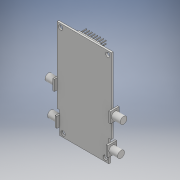
# Autodesk Inventor part: PE-43120-EVB
Saved by Autodesk Inventor 2018 (Build 220112000, 112)
## iProperties
Created: 2018-01-02
Part Number: PE-43120-EVB
Material: Generic
Document SubType Name: Modeling
Designer: rwradema
Density: 1 g/cm^3
Appearance: Default
Author: rwradema
Autodesk Inventor part; units mm, degrees
ref_plane "YZ Plane" through (0, 0, 0) normal (1, 0, 0) x (0, 1, 0)
ref_plane "XZ Plane" through (0, 0, 0) normal (0, 1, 0) x (-1, 0, 0)
ref_plane "XY Plane" through (0, 0, 0) normal (0, 0, 1) x (1, 0, 0)
sketch "Sketch1" plane through (0, 0, 0) normal (0, 1, 0) x (-1, 0, 0)
  line L0 (24.8, -18.7) -> (24.8, 50)
  line L1 (24.8, 50) -> (-24.8, 50)
  line L2 (-24.8, 50) -> (-24.8, -18.7)
  line L3 (-24.8, -18.7) -> (-22.5, -18.7)
  line L4 (-22.5, -18.7) -> (-22.5, -39)
  line L5 (-22.5, -39) -> (22.5, -39)
  line L6 (22.5, -39) -> (22.5, -18.7)
  line L7 (22.5, -18.7) -> (24.8, -18.7)
  line L8 (0, 42.3382) -> (0, -37.7046) construction
  point P0 (0, 0)
  dimension "d0" = 49.6
  dimension "d1" = 45
  dimension "d2" = 89
  dimension "d3" = 68.7
  dimension "d4" = 50
  constraints: 18 end point, 8 perpendicular, 1 collinear, 1 point on line, 1 vertical, 1 other
  measures "d0" distance of L0.end L1.end
  measures "d1" distance of L4.end L5.end
  measures "d2" distance between parallel lines of L1 L5
  measures "d3" distance of L0.start L0.end
  measures "d4" distance from line of L1 point (0, 0)
extrude "Extrusion1" add sketch "Sketch1" along normal blind 1.63
sketch "Sketch2" plane through (0, 1.63, 0) normal (0, 1, 0) x (1, 0, 0)
  circle A0 centre (-21.55, -46.75) radius 2
  circle A1 centre (21.55, -46.75) radius 2
  circle A2 centre (19.25, 35.75) radius 2
  circle A3 centre (-19.25, 35.75) radius 2
  line L0 (-24.8, 18.7) -> (-24.8, -50) projected
  line L1 (-24.8, -50) -> (24.8, -50) projected
  line L2 (22.5, 39) -> (-22.5, 39) projected
  line L3 (22.5, 18.7) -> (22.5, 39) projected
  line L4 (-22.5, 39) -> (-22.5, 18.7) projected
  point P0 (0, 0)
  dimension "d7" = 4
  dimension "d8" = 3.25
  dimension "d9" = 3.25
  dimension "d10" = 3.25
  dimension "d11" = 3.25
  dimension "d12" = 3.25
  dimension "d13" = 3.25
  dimension "d14" = 3.25
  dimension "d15" = 3.25
  constraints: 4 centre point, 3 equal radius
  measures "d7" diameter of A3
  measures "d8" distance from line of L0 A0.centre
  measures "d9" distance from line of L1 A0.centre
  measures "d10" horizontal distance of L1.end A1.centre
  measures "d11" distance from line of L1 A1.centre
  measures "d12" distance from line of A2.centre L2
  measures "d13" distance from line of L3 A2.centre
  measures "d14" distance from line of L2 A3.centre
  measures "d15" distance from line of L4 A3.centre
extrude "Extrusion2" cut sketch "Sketch2" against normal up to next
sketch "Sketch3" plane through (24.8, 0, 50) normal (1, 0, 0) x (0, 0, -1)
  line L0 (44.7, 5.63) -> (54.3, 5.63)
  line L1 (54.3, 5.63) -> (54.3, -2.37)
  line L2 (54.3, -2.37) -> (44.7, -2.37)
  line L3 (44.7, -2.37) -> (44.7, 5.63)
  line L4 (0, 1.63) -> (68.7, 1.63) projected
  line L5 (44.7, 5.63) -> (54.3, -2.37) construction
  line L6 (54.3, 5.63) -> (44.7, -2.37) construction
  line L7 (0, 0) -> (0, 1.63) projected
  point P0 (50, 0)
  point P1 (49.5, 1.63)
  dimension "d18" = 9.6
  dimension "d19" = 8
  dimension "d20" = 49.5
  constraints: 12 end point, 2 midpoint, 2 parallel, 1 horizontal, 1 perpendicular, 1 point on line
  measures "d18" distance of L0.start L0.end
  measures "d19" distance of L2.end L0.start
  measures "d20" distance from line of L7 point (49.5, 1.63)
extrude "Extrusion3" add sketch "Sketch3" along normal blind 1.5
sketch "Sketch4" plane through (22.5, 0, -18.7) normal (1, 0, 0) x (0, 0, -1)
  line L0 (4, 5.63) -> (13.6, 5.63)
  line L1 (13.6, 5.63) -> (13.6, -2.37)
  line L2 (13.6, -2.37) -> (4, -2.37)
  line L3 (4, -2.37) -> (4, 5.63)
  line L4 (20.3, 1.63) -> (0, 1.63) projected
  line L5 (4, 5.63) -> (13.6, -2.37) construction
  line L6 (13.6, 5.63) -> (4, -2.37) construction
  point P0 (-18.7, 0)
  point P1 (8.8, 1.63)
  dimension "d23" = 9.6
  dimension "d24" = 8
  dimension "d25" = 11.5
  constraints: 12 end point, 2 midpoint, 2 parallel, 1 horizontal, 1 perpendicular, 1 point on line
  measures "d23" distance of L0.start L0.end
  measures "d24" distance of L0.end L1.end
  measures "d25" distance of L4.start point (8.8, 1.63)
extrude "Extrusion4" add sketch "Sketch4" along normal blind 1.5
sketch "Sketch5" plane through (26.3, 0, 50) normal (1, 0, 0) x (0, 0, -1)
  line L0 (44.7, 5.63) -> (54.3, 5.63) construction
  line L1 (49.5, 5.63) -> (49.5, -2.37) construction
  line L2 (54.3, -2.37) -> (44.7, -2.37) construction
  line L3 (44.7, 1.63) -> (54.3, 1.63) construction
  line L4 (44.7, 1.63) -> (54.3, 1.63) construction
  circle A0 centre (49.5, 1.63) radius 3.15
  point P0 (50, 0)
  dimension "d28" = 6.3
  constraints: 4 end point, 3 midpoint, 1 centre point, 1 collinear
  measures "d28" diameter of A0
sketch "Sketch6" plane through (24, 0, -18.7) normal (1, 0, 0) x (0, 0, -1)
  line L0 (13.6, 5.63) -> (4, 5.63) construction
  line L1 (8.8, 5.63) -> (8.8, -2.37) construction
  line L2 (4, -2.37) -> (13.6, -2.37) construction
  line L3 (13.6, -2.37) -> (13.6, 5.63) construction
  line L4 (4, 0) -> (4, 1.63) construction
  line L5 (13.6, 1.63) -> (4, 1.63) construction
  circle A0 centre (8.8, 1.63) radius 3.15
  point P0 (-18.7, 0)
  dimension "d29" = 6.3
  constraints: 4 end point, 4 midpoint, 1 centre point, 1 perpendicular
  measures "d29" diameter of A0
extrude "Extrusion5" add sketch "Sketch6" along normal blind 8
extrude "Extrusion6" add sketch "Sketch5" along normal blind 8
mirror "Mirror1" about plane through (0, 0, 0) normal (1, 0, 0) of "Extrusion5", "Extrusion6", "Extrusion4", "Extrusion3"
sketch "Sketch7" plane through (0, 1.63, 0) normal (0, 1, 0) x (1, 0, 0)
  line L0 (-9.2, -48.75) -> (11.38, -48.75)
  line L1 (11.38, -48.75) -> (11.38, -43.67)
  line L2 (11.38, -43.67) -> (-9.2, -43.67)
  line L3 (-9.2, -43.67) -> (-9.2, -48.75)
  line L4 (-9.2, -48.75) -> (11.38, -43.67) construction
  line L5 (11.38, -48.75) -> (-9.2, -43.67) construction
  line L6 (-24.8, -50) -> (24.8, -50) projected
  line L7 (24.8, -50) -> (24.8, -5.3) projected
  line L8 (-24.8, -5.3) -> (-24.8, -50) projected
  point P0 (0, 0)
  point P1 (1.09, -46.21)
  dimension "d34" = 20.58
  dimension "d35" = 5.08
  dimension "d36" = 1.25
  dimension "d38" = 15.6
  constraints: 12 end point, 2 midpoint, 2 parallel, 1 horizontal, 1 perpendicular
  measures "d34" distance of L1.end L2.end
  measures "d35" distance of L2.end L0.start
  measures "d36" distance between parallel lines of L6 L0
  measures "d38" distance between parallel lines of L8 L3
extrude "Extrusion7" add sketch "Sketch7" along normal blind 2.4
sketch "Sketch8" plane through (0, 4.03, 0) normal (0, 1, 0) x (1, 0, 0)
  line L0 (10.37, -47.74) -> (9.73, -47.74)
  line L1 (9.73, -47.74) -> (9.73, -47.1)
  line L2 (9.73, -47.1) -> (10.37, -47.1)
  line L3 (10.37, -47.1) -> (10.37, -47.74)
  line L4 (10.37, -47.74) -> (9.73, -47.1) construction
  line L5 (9.73, -47.74) -> (10.37, -47.1) construction
  line L6 (11.38, -48.75) -> (11.38, -43.67) projected
  line L7 (-9.2, -48.75) -> (11.38, -48.75) projected
  line L8 (7.19, -47.74) -> (7.19, -47.1)
  line L9 (7.83, -47.74) -> (7.19, -47.74)
  line L10 (7.83, -47.1) -> (7.83, -47.74)
  line L11 (7.19, -47.1) -> (7.83, -47.1)
  line L12 (4.65, -47.74) -> (4.65, -47.1)
  line L13 (5.29, -47.74) -> (4.65, -47.74)
  line L14 (5.29, -47.1) -> (5.29, -47.74)
  line L15 (4.65, -47.1) -> (5.29, -47.1)
  line L16 (2.11, -47.74) -> (2.11, -47.1)
  line L17 (2.75, -47.74) -> (2.11, -47.74)
  line L18 (2.75, -47.1) -> (2.75, -47.74)
  line L19 (2.11, -47.1) -> (2.75, -47.1)
  line L20 (-0.43, -47.74) -> (-0.43, -47.1)
  line L21 (0.21, -47.74) -> (-0.43, -47.74)
  line L22 (0.21, -47.1) -> (0.21, -47.74)
  line L23 (-0.43, -47.1) -> (0.21, -47.1)
  line L24 (-2.97, -47.74) -> (-2.97, -47.1)
  line L25 (-2.33, -47.74) -> (-2.97, -47.74)
  line L26 (-2.33, -47.1) -> (-2.33, -47.74)
  line L27 (-2.97, -47.1) -> (-2.33, -47.1)
  line L28 (-5.51, -47.74) -> (-5.51, -47.1)
  line L29 (-4.87, -47.74) -> (-5.51, -47.74)
  line L30 (-4.87, -47.1) -> (-4.87, -47.74)
  line L31 (-5.51, -47.1) -> (-4.87, -47.1)
  line L32 (-8.05, -47.74) -> (-8.05, -47.1)
  line L33 (-7.41, -47.74) -> (-8.05, -47.74)
  line L34 (-7.41, -47.1) -> (-7.41, -47.74)
  line L35 (-8.05, -47.1) -> (-7.41, -47.1)
  line L36 (9.73, -45.2) -> (9.73, -44.56)
  line L37 (10.37, -45.2) -> (9.73, -45.2)
  line L38 (10.37, -44.56) -> (10.37, -45.2)
  line L39 (9.73, -44.56) -> (10.37, -44.56)
  line L40 (7.19, -45.2) -> (7.19, -44.56)
  line L41 (7.83, -45.2) -> (7.19, -45.2)
  line L42 (7.83, -44.56) -> (7.83, -45.2)
  line L43 (7.19, -44.56) -> (7.83, -44.56)
  line L44 (4.65, -45.2) -> (4.65, -44.56)
  line L45 (5.29, -45.2) -> (4.65, -45.2)
  line L46 (5.29, -44.56) -> (5.29, -45.2)
  line L47 (4.65, -44.56) -> (5.29, -44.56)
  line L48 (2.11, -45.2) -> (2.11, -44.56)
  line L49 (2.75, -45.2) -> (2.11, -45.2)
  line L50 (2.75, -44.56) -> (2.75, -45.2)
  line L51 (2.11, -44.56) -> (2.75, -44.56)
  line L52 (-0.43, -45.2) -> (-0.43, -44.56)
  line L53 (0.21, -45.2) -> (-0.43, -45.2)
  line L54 (0.21, -44.56) -> (0.21, -45.2)
  line L55 (-0.43, -44.56) -> (0.21, -44.56)
  line L56 (-2.97, -45.2) -> (-2.97, -44.56)
  line L57 (-2.33, -45.2) -> (-2.97, -45.2)
  line L58 (-2.33, -44.56) -> (-2.33, -45.2)
  line L59 (-2.97, -44.56) -> (-2.33, -44.56)
  line L60 (-5.51, -45.2) -> (-5.51, -44.56)
  line L61 (-4.87, -45.2) -> (-5.51, -45.2)
  line L62 (-4.87, -44.56) -> (-4.87, -45.2)
  line L63 (-5.51, -44.56) -> (-4.87, -44.56)
  line L64 (-8.05, -45.2) -> (-8.05, -44.56)
  line L65 (-7.41, -45.2) -> (-8.05, -45.2)
  line L66 (-7.41, -44.56) -> (-7.41, -45.2)
  line L67 (-8.05, -44.56) -> (-7.41, -44.56)
  point P0 (0, 0)
  point P1 (10.05, -47.42)
  dimension "d41" = 0.64
  dimension "d42" = 1.65
  dimension "d43" = 1.65
  dimension "d46" = 2.54
  dimension "d49" = 2.54
  constraints: 132 end point, 2 horizontal, 2 midpoint, 2 parallel, 2 perpendicular, 1 vertical, 120 other
  measures "d41" distance of L2.end L0.start
  measures "d42" distance between parallel lines of L6 L1
  measures "d43" distance between parallel lines of L7 L2
  measures "d46" distance of L0.end L8.start
  measures "d49" distance of L0.end L36.start
extrude "Extrusion8" add sketch "Sketch8" along normal blind 5.76
sketch "Sketch9" plane through (0, 1.63, 0) normal (0, 1, 0) x (1, 0, 0)
  line L0 (5.9, 14.8) -> (8.44, 14.8)
  line L1 (8.44, 14.8) -> (8.44, 19.88)
  line L2 (8.44, 19.88) -> (5.9, 19.88)
  line L3 (5.9, 19.88) -> (5.9, 14.8)
  line L4 (5.9, 14.8) -> (8.44, 19.88) construction
  line L5 (8.44, 14.8) -> (5.9, 19.88) construction
  line L6 (22.5, 18.7) -> (22.5, 22.7) projected
  line L7 (22.5, 39) -> (-22.5, 39) projected
  point P0 (0, 0)
  point P1 (7.17, 17.34)
  dimension "d54" = 5.08
  dimension "d55" = 2.54
  dimension "d56" = 16.6
  dimension "d57" = 24.2
  constraints: 12 end point, 2 midpoint, 2 parallel, 1 horizontal, 1 perpendicular
  measures "d54" distance of L2.end L0.start
  measures "d55" distance of L0.start L0.end
  measures "d56" distance between parallel lines of L6 L3
  measures "d57" distance between parallel lines of L7 L0
extrude "Extrusion9" add sketch "Sketch9" along normal blind 11.3
body "Solid1"
